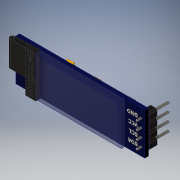
# Autodesk Inventor part: Part1
Saved by Autodesk Inventor 2019 (Build 230136000, 136)
## iProperties
Created: 2025-05-31
Part Number: Part1
Material: Generic
Document SubType Name: Modeling
Designer: Zide
Density: 1 g/cm^3
Appearance: Default
Author: Zide
Autodesk Inventor part; units mm, degrees
(part 1 of 4)
ref_plane "YZ Plane" through (0, 0, 0) normal (1, 0, 0) x (0, 1, 0)
ref_plane "XZ Plane" through (0, 0, 0) normal (0, 1, 0) x (-1, 0, 0)
ref_plane "XY Plane" through (0, 0, 0) normal (0, 0, 1) x (1, 0, 0)
sketch "Sketch1" plane through (0, 0, 0) normal (0, 0, 1) x (1, 0, 0)
  line L0 (-18.8, 6.05) -> (18.8, 6.05)
  line L1 (18.8, -6.05) -> (-18.8, -6.05)
  line L2 (-18.8, -6.05) -> (-18.8, 6.05)
  line L3 (-18.8, 6.05) -> (18.8, -6.05) construction
  line L4 (18.8, 6.05) -> (-18.8, -6.05) construction
  line L5 (-18.8, 0) -> (18.8, 0)
  line L6 (0, 6.05) -> (0, -6.05)
  line L7 (18.8, 3.63) -> (17.8, 3.63)
  line L8 (17.95, 3.38) -> (17.65, 3.38)
  line L9 (17.55, 3.48) -> (17.55, 3.78)
  line L10 (17.65, 3.88) -> (17.95, 3.88)
  line L11 (18.05, 3.78) -> (18.05, 3.48)
  line L12 (18.05, 3.38) -> (17.55, 3.88) construction
  line L13 (17.55, 3.38) -> (18.05, 3.88) construction
  line L14 (17.55, 3.78) -> (17.65, 3.88)
  line L15 (17.95, 3.88) -> (18.05, 3.78)
  line L16 (18.05, 3.48) -> (17.95, 3.38)
  line L17 (17.55, 3.48) -> (17.65, 3.38)
  line L18 (18.8, 1.21) -> (17.8, 1.21)
  line L19 (17.95, 0.96) -> (17.65, 0.96)
  line L20 (17.55, 1.06) -> (17.55, 1.36)
  line L21 (17.65, 1.46) -> (17.95, 1.46)
  line L22 (18.05, 1.36) -> (18.05, 1.06)
  line L23 (18.05, 0.96) -> (17.55, 1.46) construction
  line L24 (17.55, 0.96) -> (18.05, 1.46) construction
  line L25 (17.55, 1.36) -> (17.65, 1.46)
  line L26 (17.95, 1.46) -> (18.05, 1.36)
  line L27 (18.05, 1.06) -> (17.95, 0.96)
  line L28 (17.55, 1.06) -> (17.65, 0.96)
  line L29 (18.8, -1.21) -> (17.8, -1.21)
  line L30 (17.95, -1.46) -> (17.65, -1.46)
  line L31 (17.55, -1.36) -> (17.55, -1.06)
  line L32 (17.65, -0.96) -> (17.95, -0.96)
  line L33 (18.05, -1.06) -> (18.05, -1.36)
  line L34 (18.05, -1.46) -> (17.55, -0.96) construction
  line L35 (17.55, -1.46) -> (18.05, -0.96) construction
  line L36 (17.55, -1.06) -> (17.65, -0.96)
  line L37 (17.95, -0.96) -> (18.05, -1.06)
  line L38 (18.05, -1.36) -> (17.95, -1.46)
  line L39 (17.55, -1.36) -> (17.65, -1.46)
  line L40 (18.8, -3.63) -> (17.8, -3.63)
  line L41 (17.95, -3.88) -> (17.65, -3.88)
  line L42 (17.55, -3.78) -> (17.55, -3.48)
  line L43 (17.65, -3.38) -> (17.95, -3.38)
  line L44 (18.05, -3.48) -> (18.05, -3.78)
  line L45 (18.05, -3.88) -> (17.55, -3.38) construction
  line L46 (17.55, -3.88) -> (18.05, -3.38) construction
  line L47 (17.55, -3.48) -> (17.65, -3.38)
  line L48 (17.95, -3.38) -> (18.05, -3.48)
  line L49 (18.05, -3.78) -> (17.95, -3.88)
  line L50 (17.55, -3.78) -> (17.65, -3.88)
  line L51 (18.8, 3.63) -> (18.8, 1.21)
  line L52 (18.8, 1.21) -> (18.8, -1.21)
  line L53 (18.8, -1.21) -> (18.8, -3.63)
  line L54 (18.8, -6.05) -> (18.8, -3.63)
  line L55 (18.8, 3.63) -> (18.8, 6.05)
  point P0 (0, 0)
  dimension "d0" = 37.6
  dimension "d1" = 12.1
  constraints: 112 end point, 32 point on line, 13 midpoint, 12 equal length, 9 horizontal, 4 perpendicular, 2 vertical
  measures "d0" distance of L0.start L0.end
  measures "d1" distance of L0.end L1.start
extrude "Extrusion1" add sketch "Sketch1" along normal blind 1.1
sketch "Sketch2" plane through (0, 0, 0) normal (0, 0, -1) x (-1, 0, 0)
  line L0 (-17.65, -3.88) -> (-17.95, -3.88)
  line L1 (-17.95, -3.88) -> (-18.05, -3.78)
  line L2 (-18.05, -3.78) -> (-18.05, -3.48)
  line L3 (-18.05, -3.48) -> (-17.95, -3.38)
  line L4 (-17.95, -3.38) -> (-17.65, -3.38)
  line L5 (-17.65, -3.38) -> (-17.55, -3.48)
  line L6 (-17.55, -3.48) -> (-17.55, -3.78)
  line L7 (-17.55, -3.78) -> (-17.65, -3.88)
  line L8 (-17.65, -1.46) -> (-17.95, -1.46)
  line L9 (-17.95, -1.46) -> (-18.05, -1.36)
  line L10 (-18.05, -1.36) -> (-18.05, -1.06)
  line L11 (-18.05, -1.06) -> (-17.95, -0.96)
  line L12 (-17.95, -0.96) -> (-17.65, -0.96)
  line L13 (-17.65, -0.96) -> (-17.55, -1.06)
  line L14 (-17.55, -1.06) -> (-17.55, -1.36)
  line L15 (-17.55, -1.36) -> (-17.65, -1.46)
  line L16 (-17.65, 0.96) -> (-17.95, 0.96)
  line L17 (-17.95, 0.96) -> (-18.05, 1.06)
  line L18 (-18.05, 1.06) -> (-18.05, 1.36)
  line L19 (-18.05, 1.36) -> (-17.95, 1.46)
  line L20 (-17.95, 1.46) -> (-17.65, 1.46)
  line L21 (-17.65, 1.46) -> (-17.55, 1.36)
  line L22 (-17.55, 1.36) -> (-17.55, 1.06)
  line L23 (-17.55, 1.06) -> (-17.65, 0.96)
  line L24 (-17.95, 3.88) -> (-17.65, 3.88)
  line L25 (-17.65, 3.88) -> (-17.55, 3.78)
  line L26 (-17.55, 3.78) -> (-17.55, 3.48)
  line L27 (-17.55, 3.48) -> (-17.65, 3.38)
  line L28 (-17.65, 3.38) -> (-17.95, 3.38)
  line L29 (-17.95, 3.38) -> (-18.05, 3.48)
  line L30 (-18.05, 3.48) -> (-18.05, 3.78)
  line L31 (-18.05, 3.78) -> (-17.95, 3.88)
  line L32 (-18.8, 6.05) -> (18.8, 6.05)
  line L33 (18.8, -6.05) -> (-18.8, -6.05)
  line L34 (18.8, 6.05) -> (18.8, -6.05)
  line L35 (-17.65, 3.38) -> (-17.95, 3.38)
  line L36 (-18.05, 3.78) -> (-18.05, 3.48)
  line L37 (-17.55, 3.48) -> (-17.55, 3.78)
  line L38 (-16.6, -4.33) -> (-16.6, -2.93)
  line L39 (-19, -2.93) -> (-19, -4.33)
  line L40 (-18.5, -4.83) -> (-17.1, -4.83)
  line L41 (-19, -2.93) -> (-18.5, -2.43)
  line L42 (-17.1, -2.43) -> (-16.6, -2.93)
  line L43 (-16.6, -4.33) -> (-17.1, -4.83)
  line L44 (-18.5, -4.83) -> (-19, -4.33)
  line L45 (-16.6, -1.91) -> (-16.6, -0.51)
  line L46 (-19, -0.51) -> (-19, -1.91)
  line L47 (-19, -0.51) -> (-18.5, -0.01)
  line L48 (-17.1, -0.01) -> (-16.6, -0.51)
  line L49 (-16.6, -1.91) -> (-17.1, -2.41)
  line L50 (-18.5, -2.41) -> (-19, -1.91)
  line L51 (-19, 1.91) -> (-18.5, 2.41)
  line L52 (-17.1, 2.41) -> (-16.6, 1.91)
  line L53 (-16.6, 0.51) -> (-16.6, 1.91)
  line L54 (-19, 1.91) -> (-19, 0.51)
  line L55 (-16.6, 0.51) -> (-17.1, 0.01)
  line L56 (-18.5, 0.01) -> (-19, 0.51)
  line L57 (-17.95, 3.88) -> (-17.65, 3.88)
  line L58 (-19, 4.33) -> (-19, 2.93)
  line L59 (-16.6, 2.93) -> (-16.6, 4.33)
  line L60 (-17.1, 4.83) -> (-16.6, 4.33)
  line L61 (-17.1, 4.83) -> (-18.5, 4.83)
  line L62 (-19, 4.33) -> (-18.5, 4.83)
  line L63 (-16.6, 2.93) -> (-17.1, 2.43)
  line L64 (-18.5, 2.43) -> (-19, 2.93)
  line L65 (-18.5, -2.41) -> (-18.5, -2.43)
  line L66 (-17.1, -2.43) -> (-17.1, -2.41)
  line L67 (-18.5, -0.01) -> (-18.5, 0.01)
  line L68 (-17.1, -0.01) -> (-17.1, 0.01)
  line L69 (-18.5, 2.41) -> (-18.5, 2.43)
  line L70 (-17.1, 2.41) -> (-17.1, 2.43)
  point P0 (0, 0)
  constraints: 64 end point, 5 parallel, 5 vertical, 1 perpendicular
extrude "Extrusion2" add sketch "Sketch2" along normal blind 2.3 separate body
sketch "Sketch3" plane through (0, 0, 1.1) normal (0, 0, 1) x (1, 0, 0)
  line L0 (17.95, -3.88) -> (17.65, -3.88)
  line L1 (17.65, -3.88) -> (17.55, -3.78)
  line L2 (17.55, -3.78) -> (17.55, -3.48)
  line L3 (17.55, -3.48) -> (17.65, -3.38)
  line L4 (17.65, -3.38) -> (17.95, -3.38)
  line L5 (17.95, -3.38) -> (18.05, -3.48)
  line L6 (18.05, -3.48) -> (18.05, -3.78)
  line L7 (18.05, -3.78) -> (17.95, -3.88)
  line L8 (17.95, -1.46) -> (17.65, -1.46)
  line L9 (17.65, -1.46) -> (17.55, -1.36)
  line L10 (17.55, -1.36) -> (17.55, -1.06)
  line L11 (17.55, -1.06) -> (17.65, -0.96)
  line L12 (17.65, -0.96) -> (17.95, -0.96)
  line L13 (17.95, -0.96) -> (18.05, -1.06)
  line L14 (18.05, -1.06) -> (18.05, -1.36)
  line L15 (18.05, -1.36) -> (17.95, -1.46)
  line L16 (17.95, 0.96) -> (17.65, 0.96)
  line L17 (17.65, 0.96) -> (17.55, 1.06)
  line L18 (17.55, 1.06) -> (17.55, 1.36)
  line L19 (17.55, 1.36) -> (17.65, 1.46)
  line L20 (17.65, 1.46) -> (17.95, 1.46)
  line L21 (17.95, 1.46) -> (18.05, 1.36)
  line L22 (18.05, 1.36) -> (18.05, 1.06)
  line L23 (18.05, 1.06) -> (17.95, 0.96)
  line L24 (17.65, 3.88) -> (17.95, 3.88)
  line L25 (17.95, 3.88) -> (18.05, 3.78)
  line L26 (18.05, 3.78) -> (18.05, 3.48)
  line L27 (18.05, 3.48) -> (17.95, 3.38)
  line L28 (17.95, 3.38) -> (17.65, 3.38)
  line L29 (17.65, 3.38) -> (17.55, 3.48)
  line L30 (17.55, 3.48) -> (17.55, 3.78)
  line L31 (17.55, 3.78) -> (17.65, 3.88)
  line L32 (18.8, 6.05) -> (-18.8, 6.05)
  line L33 (-18.8, 6.05) -> (-18.8, -6.05)
  line L34 (-18.8, -6.05) -> (18.8, -6.05)
  line L35 (18.8, -6.05) -> (18.8, 6.05)
  point P0 (0, 0)
extrude "Extrusion3" add sketch "Sketch3" along normal blind 1.5 and the other way blind 8 separate body contours L0 L1 L2 L3 L4 L5 L6 L7 | L8 L9 L10 L11 L12 L13 L14 L15 | L16 L17 L18 L19 L20 L21 L22 L23 | L24 L25 L26 L27 L28 L29 L30 L31
chamfer "Chamfer1" distance 0.15 angle 45 32 edges at (18.05, -3.63, 2.6) (17.8, -3.38, 2.6) (17.55, -3.63, 2.6) (17.8, -3.88, 2.6) (18.05, -1.21, 2.6) (17.8, -0.96, 2.6) (17.55, -1.21, 2.6) (17.8, -1.46, 2.6) (18.05, 1.21, 2.6) (17.8, 0.96, 2.6) (17.55, 1.21, 2.6) (17.8, 1.46, 2.6) (17.8, 3.38, 2.6) (18.05, 3.63, 2.6) (17.8, 3.88, 2.6) (17.55, 3.63, 2.6) (17.8, -3.88, -6.9) (18.05, -3.63, -6.9) (17.8, -3.38, -6.9) (17.55, -3.63, -6.9) (17.8, -1.46, -6.9) (17.55, -1.21, -6.9) (17.8, -0.96, -6.9) (18.05, -1.21, -6.9) (17.8, 0.96, -6.9) (17.55, 1.21, -6.9) (17.8, 1.46, -6.9) (18.05, 1.21, -6.9) (17.8, 3.38, -6.9) (17.55, 3.63, -6.9) (17.8, 3.88, -6.9) (18.05, 3.63, -6.9)
sketch "Sketch4" plane through (0, 0, 1.1) normal (0, 0, 1) x (1, 0, 0)
  line L0 (18.8, -6.05) -> (18.8, 6.05)
  line L1 (13, -6.05) -> (13, 6.05)
  line L2 (-14.5, -6.05) -> (-14.5, 6.05)
  line L3 (-11.5, -6.05) -> (-11.5, 6.05)
  line L4 (13, -6.05) -> (-11.5, -6.05)
  line L5 (-11.5, 6.05) -> (13, 6.05)
  line L6 (18.8, 6.05) -> (-18.8, 6.05)
  point P0 (0, 0)
  dimension "d45" = 5.8
  dimension "d46" = 27.5
  dimension "d47" = 3
  constraints: 10 end point, 3 parallel, 1 collinear, 1 perpendicular
  measures "d45" distance between parallel lines of L0 L1
  measures "d46" distance between parallel lines of L1 L2
  measures "d47" distance between parallel lines of L2 L3
extrude "Extrusion4" add sketch "Sketch4" along normal blind 1.5 separate body
sketch "Sketch5" plane through (0, 0, 1.1) normal (0, 0, 1) x (1, 0, 0)
  line L0 (-11.5, 6.05) -> (-11.5, -6.05)
  line L1 (-14.5, 6.05) -> (-14.5, -6.05)
  line L2 (-11.5, -6.05) -> (-14.5, -6.05)
  line L3 (-18.8, -6.05) -> (18.8, -6.05)
  line L4 (-11.5, 6.05) -> (-14.5, 6.05)
  line L5 (18.8, 6.05) -> (-18.8, 6.05)
  point P0 (0, 0)
  dimension "d50" = 3
  constraints: 6 end point, 2 collinear, 1 parallel
  measures "d50" distance between parallel lines of L0 L1
extrude "Extrusion5" add sketch "Sketch5" along normal blind 1.5 separate body
chamfer "Chamfer2" distance 0.5 angle 45 3 edges at (0.75, -6.05, 2.6) (13, 0, 2.6) (0.75, 6.05, 2.6)
sketch "Sketch6" plane through (0, 0, 1.1) normal (0, 0, 1) x (1, 0, 0)
  line L0 (17.55, 3.78) -> (17.55, 3.48)
  line L1 (17.55, 1.36) -> (17.55, 1.06)
  line L2 (17.55, -1.06) -> (17.55, -1.36)
  line L3 (17.55, -3.48) -> (17.55, -3.78)
  line L4 (17.55, -3.48) -> (17.55, -3.78)
  line L5 (17.55, -3.63) -> (16.85, -3.63)
  line L6 (16.819, -4.1169) -> (13.9568, -4.1169) construction
  line L7 (13.9568, -4.1169) -> (13.9568, -3.0812) construction
  line L8 (13.9568, -3.0812) -> (16.819, -3.0812) construction
  line L9 (16.819, -3.0812) -> (16.819, -4.1169) construction
  line L10 (17.55, -1.21) -> (16.85, -1.21)
  line L11 (17.55, 1.21) -> (16.85, 1.21)
  line L12 (17.55, 3.63) -> (16.85, 3.63)
  line L13 (16.8164, -1.7403) -> (14.2403, -1.7403) construction
  line L14 (14.2403, -1.7403) -> (14.2403, -0.7014) construction
  line L15 (14.2403, -0.7014) -> (16.8164, -0.7014) construction
  line L16 (16.8164, -0.7014) -> (16.8164, -1.7403) construction
  line L17 (16.8624, 0.6623) -> (14.0982, 0.6623) construction
  line L18 (14.0982, 0.6623) -> (14.0982, 1.7012) construction
  line L19 (14.0982, 1.7012) -> (16.8624, 1.7012) construction
  line L20 (16.8624, 1.7012) -> (16.8624, 0.6623) construction
  line L21 (16.8549, 3.1406) -> (13.7293, 3.1406) construction
  line L22 (13.7293, 3.1406) -> (13.7293, 4.1811) construction
  line L23 (13.7293, 4.1811) -> (16.8549, 4.1811) construction
  line L24 (16.8549, 4.1811) -> (16.8549, 3.1406) construction
  spline S0 degree 2 poles (16.4065, -3.0812) (16.5216, -3.0812) (16.695, -3.1258) (16.7696, -3.1582) knots 0 0 0 1 2 2 2
  line L25 (16.7696, -3.1582) -> (16.7696, -3.3965)
  line L26 (16.7696, -3.3965) -> (16.7469, -3.3965)
  spline S1 degree 2 poles (16.7469, -3.3965) (16.6715, -3.3325) (16.4908, -3.2636) (16.4057, -3.2636) knots 0 0 0 1 2 2 2
  spline S2 degree 2 poles (16.4057, -3.2636) (16.3838, -3.2636) (16.3133, -3.2733) (16.2923, -3.283) knots 0 0 0 1 2 2 2
  spline S3 degree 2 poles (16.2923, -3.283) (16.2663, -3.2944) (16.2299, -3.3357) (16.2299, -3.3689) knots 0 0 0 1 2 2 2
  spline S4 degree 2 poles (16.2299, -3.3689) (16.2299, -3.407) (16.289, -3.454) (16.3295, -3.4645) knots 0 0 0 1 2 2 2
  spline S5 degree 2 poles (16.3295, -3.4645) (16.3806, -3.4783) (16.4965, -3.5018) (16.5475, -3.5196) knots 0 0 0 1 2 2 2
  spline S6 degree 2 poles (16.5475, -3.5196) (16.6634, -3.5602) (16.7639, -3.6987) (16.7639, -3.8025) knots 0 0 0 1 2 2 2
  spline S7 degree 2 poles (16.7639, -3.8025) (16.7639, -3.9427) (16.5265, -4.1169) (16.3482, -4.1169) knots 0 0 0 1 2 2 2
  spline S8 degree 2 poles (16.3482, -4.1169) (16.259, -4.1169) (16.0824, -4.0804) (16.0127, -4.0496) knots 0 0 0 1 2 2 2
  line L27 (16.0127, -4.0496) -> (16.0127, -3.8211)
  line L28 (16.0127, -3.8211) -> (16.0346, -3.8211)
  spline S9 degree 2 poles (16.0346, -3.8211) (16.0905, -3.8689) (16.2509, -3.9346) (16.3352, -3.9346) knots 0 0 0 1 2 2 2
  spline S10 degree 2 poles (16.3352, -3.9346) (16.3684, -3.9346) (16.4203, -3.9248) (16.4495, -3.9119) knots 0 0 0 1 2 2 2
  spline S11 degree 2 poles (16.4495, -3.9119) (16.473, -3.9013) (16.507, -3.8592) (16.507, -3.8333) knots 0 0 0 1 2 2 2
  spline S12 degree 2 poles (16.507, -3.8333) (16.507, -3.7944) (16.4527, -3.7498) (16.3749, -3.732) knots 0 0 0 1 2 2 2
  spline S13 degree 2 poles (16.3749, -3.732) (16.3247, -3.7206) (16.2315, -3.6987) (16.178, -3.6801) knots 0 0 0 1 2 2 2
  spline S14 degree 2 poles (16.178, -3.6801) (16.0743, -3.642) (15.973, -3.5156) (15.973, -3.4119) knots 0 0 0 1 2 2 2
  spline S15 degree 2 poles (15.973, -3.4119) (15.973, -3.2628) (16.2072, -3.0812) (16.4065, -3.0812) knots 0 0 0 1 2 2 2
  spline S16 degree 2 poles (14.9519, -3.5983) (14.9519, -3.4581) (15.0743, -3.2376) (15.1675, -3.1785) knots 0 0 0 1 2 2 2
  spline S17 degree 2 poles (15.1675, -3.1785) (15.2453, -3.1282) (15.4284, -3.0991) (15.5313, -3.0991) knots 0 0 0 1 2 2 2
  line L29 (15.5313, -3.0991) -> (15.8441, -3.0991)
  line L30 (15.8441, -3.0991) -> (15.8441, -4.0991)
  line L31 (15.8441, -4.0991) -> (15.5346, -4.0991)
  spline S18 degree 2 poles (15.5346, -4.0991) (15.4292, -4.0991) (15.2453, -4.0723) (15.1642, -4.0205) knots 0 0 0 1 2 2 2
  spline S19 degree 2 poles (15.1642, -4.0205) (15.0662, -3.9572) (14.9519, -3.7433) (14.9519, -3.5983) knots 0 0 0 1 2 2 2
  spline S20 degree 2 poles (15.2096, -3.5999) (15.2096, -3.6987) (15.2777, -3.8397) (15.3474, -3.8795) knots 0 0 0 1 2 2 2
  spline S21 degree 2 poles (15.3474, -3.8795) (15.3984, -3.907) (15.5103, -3.9127) (15.588, -3.9127) knots 0 0 0 1 2 2 2
  line L32 (15.588, -3.9127) -> (15.5929, -3.9127)
  line L33 (15.5929, -3.9127) -> (15.5929, -3.2863)
  line L34 (15.5929, -3.2863) -> (15.588, -3.2863)
  spline S22 degree 2 poles (15.588, -3.2863) (15.5038, -3.2863) (15.3879, -3.2919) (15.3352, -3.3252) knots 0 0 0 1 2 2 2
  spline S23 degree 2 poles (15.3352, -3.3252) (15.2736, -3.3641) (15.2096, -3.501) (15.2096, -3.5999) knots 0 0 0 1 2 2 2
  line L35 (14.9106, -3.0991) -> (14.5727, -4.0991)
  line L36 (14.5727, -4.0991) -> (14.2987, -4.0991)
  line L37 (14.2987, -4.0991) -> (13.9608, -3.0991)
  line L38 (13.9608, -3.0991) -> (14.2193, -3.0991)
  line L39 (14.2193, -3.0991) -> (14.2817, -3.3033)
  line L40 (14.2817, -3.3033) -> (14.5962, -3.3033)
  line L41 (14.5962, -3.3033) -> (14.6594, -3.0991)
  line L42 (14.6594, -3.0991) -> (14.9106, -3.0991)
  line L43 (14.3368, -3.4848) -> (14.4389, -3.8154)
  line L44 (14.4389, -3.8154) -> (14.5419, -3.4848)
  line L45 (14.5419, -3.4848) -> (14.3368, -3.4848)
  spline S24 degree 2 poles (16.404, -0.703) (16.519, -0.703) (16.6925, -0.7476) (16.767, -0.78) knots 0 0 0 1 2 2 2
  line L46 (16.767, -0.78) -> (16.767, -1.0183)
  line L47 (16.767, -1.0183) -> (16.7443, -1.0183)
  spline S25 degree 2 poles (16.7443, -1.0183) (16.669, -0.9543) (16.4882, -0.8854) (16.4032, -0.8854) knots 0 0 0 1 2 2 2
  spline S26 degree 2 poles (16.4032, -0.8854) (16.3813, -0.8854) (16.3108, -0.8951) (16.2897, -0.9048) knots 0 0 0 1 2 2 2
  spline S27 degree 2 poles (16.2897, -0.9048) (16.2638, -0.9162) (16.2273, -0.9575) (16.2273, -0.9907) knots 0 0 0 1 2 2 2
  spline S28 degree 2 poles (16.2273, -0.9907) (16.2273, -1.0288) (16.2865, -1.0758) (16.327, -1.0863) knots 0 0 0 1 2 2 2
  spline S29 degree 2 poles (16.327, -1.0863) (16.378, -1.1001) (16.4939, -1.1236) (16.545, -1.1415) knots 0 0 0 1 2 2 2
  spline S30 degree 2 poles (16.545, -1.1415) (16.6609, -1.182) (16.7613, -1.3205) (16.7613, -1.4243) knots 0 0 0 1 2 2 2
  spline S31 degree 2 poles (16.7613, -1.4243) (16.7613, -1.5645) (16.5239, -1.7387) (16.3456, -1.7387) knots 0 0 0 1 2 2 2
  spline S32 degree 2 poles (16.3456, -1.7387) (16.2565, -1.7387) (16.0798, -1.7022) (16.0101, -1.6714) knots 0 0 0 1 2 2 2
  line L48 (16.0101, -1.6714) -> (16.0101, -1.4429)
  line L49 (16.0101, -1.4429) -> (16.032, -1.4429)
  spline S33 degree 2 poles (16.032, -1.4429) (16.0879, -1.4907) (16.2484, -1.5564) (16.3327, -1.5564) knots 0 0 0 1 2 2 2
  spline S34 degree 2 poles (16.3327, -1.5564) (16.3659, -1.5564) (16.4177, -1.5466) (16.4469, -1.5337) knots 0 0 0 1 2 2 2
  spline S35 degree 2 poles (16.4469, -1.5337) (16.4704, -1.5231) (16.5045, -1.481) (16.5045, -1.4551) knots 0 0 0 1 2 2 2
  spline S36 degree 2 poles (16.5045, -1.4551) (16.5045, -1.4162) (16.4502, -1.3716) (16.3724, -1.3538) knots 0 0 0 1 2 2 2
  spline S37 degree 2 poles (16.3724, -1.3538) (16.3221, -1.3424) (16.2289, -1.3205) (16.1754, -1.3019) knots 0 0 0 1 2 2 2
  spline S38 degree 2 poles (16.1754, -1.3019) (16.0717, -1.2638) (15.9704, -1.1374) (15.9704, -1.0337) knots 0 0 0 1 2 2 2
  spline S39 degree 2 poles (15.9704, -1.0337) (15.9704, -0.8846) (16.2046, -0.703) (16.404, -0.703) knots 0 0 0 1 2 2 2
  spline S40 degree 2 poles (15.4104, -0.7014) (15.6357, -0.7014) (15.8999, -0.9737) (15.8999, -1.2201) knots 0 0 0 1 2 2 2
  spline S41 degree 2 poles (15.8999, -1.2201) (15.8999, -1.4575) (15.6349, -1.7403) (15.4096, -1.7403) knots 0 0 0 1 2 2 2
  spline S42 degree 2 poles (15.4096, -1.7403) (15.3505, -1.7403) (15.2549, -1.7265) (15.2111, -1.7152) knots 0 0 0 1 2 2 2
  spline S43 degree 2 poles (15.2111, -1.7152) (15.1771, -1.7047) (15.0968, -1.6698) (15.0717, -1.6568) knots 0 0 0 1 2 2 2
  line L50 (15.0717, -1.6568) -> (15.0717, -1.4186)
  line L51 (15.0717, -1.4186) -> (15.0968, -1.4186)
  spline S44 degree 2 poles (15.0968, -1.4186) (15.1155, -1.4348) (15.1706, -1.4802) (15.2054, -1.5013) knots 0 0 0 1 2 2 2
  spline S45 degree 2 poles (15.2054, -1.5013) (15.2403, -1.5231) (15.3237, -1.5531) (15.3699, -1.5531) knots 0 0 0 1 2 2 2
  spline S46 degree 2 poles (15.3699, -1.5531) (15.4242, -1.5531) (15.5142, -1.5191) (15.5555, -1.4761) knots 0 0 0 1 2 2 2
  spline S47 degree 2 poles (15.5555, -1.4761) (15.5928, -1.438) (15.6406, -1.3076) (15.6406, -1.2192) knots 0 0 0 1 2 2 2
  spline S48 degree 2 poles (15.6406, -1.2192) (15.6406, -1.1261) (15.5912, -0.9988) (15.5506, -0.9599) knots 0 0 0 1 2 2 2
  spline S49 degree 2 poles (15.5506, -0.9599) (15.5117, -0.9218) (15.4161, -0.8886) (15.3683, -0.8886) knots 0 0 0 1 2 2 2
  spline S50 degree 2 poles (15.3683, -0.8886) (15.3189, -0.8886) (15.2289, -0.9218) (15.1981, -0.9421) knots 0 0 0 1 2 2 2
  spline S51 degree 2 poles (15.1981, -0.9421) (15.1641, -0.9624) (15.113, -1.0053) (15.0944, -1.0223) knots 0 0 0 1 2 2 2
  line L52 (15.0944, -1.0223) -> (15.0717, -1.0223)
  line L53 (15.0717, -1.0223) -> (15.0717, -0.7873)
  spline S52 degree 2 poles (15.0717, -0.7873) (15.0993, -0.7744) (15.1714, -0.7419) (15.2103, -0.7306) knots 0 0 0 1 2 2 2
  spline S53 degree 2 poles (15.2103, -0.7306) (15.2573, -0.716) (15.3391, -0.7014) (15.4104, -0.7014) knots 0 0 0 1 2 2 2
  line L54 (14.2565, -0.7209) -> (14.9234, -0.7209)
  line L55 (14.9234, -0.7209) -> (14.9234, -1.7209)
  line L56 (14.9234, -1.7209) -> (14.6722, -1.7209)
  line L57 (14.6722, -1.7209) -> (14.6722, -0.9113)
  line L58 (14.6722, -0.9113) -> (14.2565, -0.9113)
  line L59 (14.2565, -0.9113) -> (14.2565, -0.7209)
  line L60 (15.924, 0.6818) -> (16.2676, 1.6818)
  line L61 (16.2676, 1.6818) -> (16.5293, 1.6818)
  line L62 (16.5293, 1.6818) -> (16.8729, 0.6818)
  line L63 (16.8729, 0.6818) -> (16.6128, 0.6818)
  line L64 (16.6128, 0.6818) -> (16.3948, 1.3601)
  line L65 (16.3948, 1.3601) -> (16.1776, 0.6818)
  line L66 (16.1776, 0.6818) -> (15.924, 0.6818)
  spline S54 degree 2 poles (15.3997, 1.7012) (15.6249, 1.7012) (15.8891, 1.4289) (15.8891, 1.1826) knots 0 0 0 1 2 2 2
  spline S55 degree 2 poles (15.8891, 1.1826) (15.8891, 0.9451) (15.6241, 0.6623) (15.3988, 0.6623) knots 0 0 0 1 2 2 2
  spline S56 degree 2 poles (15.3988, 0.6623) (15.3397, 0.6623) (15.2441, 0.6761) (15.2003, 0.6875) knots 0 0 0 1 2 2 2
  spline S57 degree 2 poles (15.2003, 0.6875) (15.1663, 0.698) (15.086, 0.7328) (15.0609, 0.7458) knots 0 0 0 1 2 2 2
  line L67 (15.0609, 0.7458) -> (15.0609, 0.984)
  line L68 (15.0609, 0.984) -> (15.086, 0.984)
  spline S58 degree 2 poles (15.086, 0.984) (15.1047, 0.9678) (15.1598, 0.9225) (15.1946, 0.9014) knots 0 0 0 1 2 2 2
  spline S59 degree 2 poles (15.1946, 0.9014) (15.2295, 0.8795) (15.3129, 0.8495) (15.3591, 0.8495) knots 0 0 0 1 2 2 2
  spline S60 degree 2 poles (15.3591, 0.8495) (15.4134, 0.8495) (15.5034, 0.8836) (15.5447, 0.9265) knots 0 0 0 1 2 2 2
  spline S61 degree 2 poles (15.5447, 0.9265) (15.582, 0.9646) (15.6298, 1.0951) (15.6298, 1.1834) knots 0 0 0 1 2 2 2
  spline S62 degree 2 poles (15.6298, 1.1834) (15.6298, 1.2766) (15.5804, 1.4038) (15.5399, 1.4427) knots 0 0 0 1 2 2 2
  spline S63 degree 2 poles (15.5399, 1.4427) (15.501, 1.4808) (15.4053, 1.514) (15.3575, 1.514) knots 0 0 0 1 2 2 2
  spline S64 degree 2 poles (15.3575, 1.514) (15.3081, 1.514) (15.2181, 1.4808) (15.1873, 1.4605) knots 0 0 0 1 2 2 2
  spline S65 degree 2 poles (15.1873, 1.4605) (15.1533, 1.4403) (15.1023, 1.3973) (15.0836, 1.3803) knots 0 0 0 1 2 2 2
  line L69 (15.0836, 1.3803) -> (15.0609, 1.3803)
  line L70 (15.0609, 1.3803) -> (15.0609, 1.6153)
  spline S66 degree 2 poles (15.0609, 1.6153) (15.0885, 1.6283) (15.1606, 1.6607) (15.1995, 1.6721) knots 0 0 0 1 2 2 2
  spline S67 degree 2 poles (15.1995, 1.6721) (15.2465, 1.6866) (15.3283, 1.7012) (15.3997, 1.7012) knots 0 0 0 1 2 2 2
  spline S68 degree 2 poles (14.4815, 1.7012) (14.7068, 1.7012) (14.971, 1.4289) (14.971, 1.1826) knots 0 0 0 1 2 2 2
  spline S69 degree 2 poles (14.971, 1.1826) (14.971, 0.9451) (14.706, 0.6623) (14.4807, 0.6623) knots 0 0 0 1 2 2 2
  spline S70 degree 2 poles (14.4807, 0.6623) (14.4215, 0.6623) (14.3259, 0.6761) (14.2822, 0.6875) knots 0 0 0 1 2 2 2
  spline S71 degree 2 poles (14.2822, 0.6875) (14.2481, 0.698) (14.1679, 0.7328) (14.1428, 0.7458) knots 0 0 0 1 2 2 2
  line L71 (14.1428, 0.7458) -> (14.1428, 0.984)
  line L72 (14.1428, 0.984) -> (14.1679, 0.984)
  spline S72 degree 2 poles (14.1679, 0.984) (14.1865, 0.9678) (14.2416, 0.9225) (14.2765, 0.9014) knots 0 0 0 1 2 2 2
  spline S73 degree 2 poles (14.2765, 0.9014) (14.3113, 0.8795) (14.3948, 0.8495) (14.441, 0.8495) knots 0 0 0 1 2 2 2
  spline S74 degree 2 poles (14.441, 0.8495) (14.4953, 0.8495) (14.5852, 0.8836) (14.6266, 0.9265) knots 0 0 0 1 2 2 2
  spline S75 degree 2 poles (14.6266, 0.9265) (14.6638, 0.9646) (14.7117, 1.0951) (14.7117, 1.1834) knots 0 0 0 1 2 2 2
  spline S76 degree 2 poles (14.7117, 1.1834) (14.7117, 1.2766) (14.6622, 1.4038) (14.6217, 1.4427) knots 0 0 0 1 2 2 2
  spline S77 degree 2 poles (14.6217, 1.4427) (14.5828, 1.4808) (14.4872, 1.514) (14.4394, 1.514) knots 0 0 0 1 2 2 2
  spline S78 degree 2 poles (14.4394, 1.514) (14.3899, 1.514) (14.3, 1.4808) (14.2692, 1.4605) knots 0 0 0 1 2 2 2
  spline S79 degree 2 poles (14.2692, 1.4605) (14.2352, 1.4403) (14.1841, 1.3973) (14.1655, 1.3803) knots 0 0 0 1 2 2 2
  line L73 (14.1655, 1.3803) -> (14.1428, 1.3803)
  line L74 (14.1428, 1.3803) -> (14.1428, 1.6153)
  spline S80 degree 2 poles (14.1428, 1.6153) (14.1703, 1.6283) (14.2424, 1.6607) (14.2813, 1.6721) knots 0 0 0 1 2 2 2
  spline S81 degree 2 poles (14.2813, 1.6721) (14.3283, 1.6866) (14.4102, 1.7012) (14.4815, 1.7012) knots 0 0 0 1 2 2 2
  spline S82 degree 2 poles (15.9165, 4.1033) (15.9821, 4.13) (16.192, 4.1811) (16.2941, 4.1811) knots 0 0 0 1 2 2 2
  spline S83 degree 2 poles (16.2941, 4.1811) (16.53, 4.1811) (16.8095, 3.9088) (16.8095, 3.6592) knots 0 0 0 1 2 2 2
  spline S84 degree 2 poles (16.8095, 3.6592) (16.8095, 3.4242) (16.53, 3.1406) (16.2868, 3.1406) knots 0 0 0 1 2 2 2
  spline S85 degree 2 poles (16.2868, 3.1406) (16.1612, 3.1406) (16.004, 3.1884) (15.9206, 3.2289) knots 0 0 0 1 2 2 2
  line L75 (15.9206, 3.2289) -> (15.9206, 3.4639)
  line L76 (15.9206, 3.4639) -> (15.9432, 3.4639)
  spline S86 degree 2 poles (15.9432, 3.4639) (15.9611, 3.4501) (16.0291, 3.3975) (16.0616, 3.3796) knots 0 0 0 1 2 2 2
  spline S87 degree 2 poles (16.0616, 3.3796) (16.0988, 3.3578) (16.1977, 3.327) (16.2528, 3.327) knots 0 0 0 1 2 2 2
  spline S88 degree 2 poles (16.2528, 3.327) (16.3168, 3.327) (16.423, 3.3675) (16.4643, 3.4088) knots 0 0 0 1 2 2 2
  spline S89 degree 2 poles (16.4643, 3.4088) (16.504, 3.4493) (16.5502, 3.5733) (16.5502, 3.6552) knots 0 0 0 1 2 2 2
  spline S90 degree 2 poles (16.5502, 3.6552) (16.5502, 3.8302) (16.3744, 3.9971) (16.2228, 3.9971) knots 0 0 0 1 2 2 2
  spline S91 degree 2 poles (16.2228, 3.9971) (16.209, 3.9971) (16.1734, 3.9955) (16.1596, 3.9947) knots 0 0 0 1 2 2 2
  line L77 (16.1596, 3.9947) -> (16.1596, 3.7978)
  line L78 (16.1596, 3.7978) -> (16.3533, 3.7978)
  line L79 (16.3533, 3.7978) -> (16.3533, 3.6106)
  line L80 (16.3533, 3.6106) -> (15.9165, 3.6106)
  line L81 (15.9165, 3.6106) -> (15.9165, 4.1033)
  line L82 (14.8703, 4.16) -> (15.1118, 4.16)
  line L83 (15.1118, 4.16) -> (15.4975, 3.4631)
  line L84 (15.4975, 3.4631) -> (15.4975, 4.16)
  line L85 (15.4975, 4.16) -> (15.7269, 4.16)
  line L86 (15.7269, 4.16) -> (15.7269, 3.16)
  line L87 (15.7269, 3.16) -> (15.4189, 3.16)
  line L88 (15.4189, 3.16) -> (15.0996, 3.733)
  line L89 (15.0996, 3.733) -> (15.0996, 3.16)
  line L90 (15.0996, 3.16) -> (14.8703, 3.16)
  line L91 (14.8703, 3.16) -> (14.8703, 4.16)
  spline S92 degree 2 poles (13.7747, 3.6608) (13.7747, 3.801) (13.8971, 4.0214) (13.9902, 4.0806) knots 0 0 0 1 2 2 2
  spline S93 degree 2 poles (13.9902, 4.0806) (14.068, 4.1308) (14.2512, 4.16) (14.3541, 4.16) knots 0 0 0 1 2 2 2
  line L92 (14.3541, 4.16) -> (14.6669, 4.16)
  line L93 (14.6669, 4.16) -> (14.6669, 3.16)
  line L94 (14.6669, 3.16) -> (14.3573, 3.16)
  spline S94 degree 2 poles (14.3573, 3.16) (14.252, 3.16) (14.068, 3.1868) (13.987, 3.2386) knots 0 0 0 1 2 2 2
  spline S95 degree 2 poles (13.987, 3.2386) (13.8889, 3.3018) (13.7747, 3.5158) (13.7747, 3.6608) knots 0 0 0 1 2 2 2
  spline S96 degree 2 poles (14.0324, 3.6592) (14.0324, 3.5603) (14.1005, 3.4193) (14.1701, 3.3796) knots 0 0 0 1 2 2 2
  spline S97 degree 2 poles (14.1701, 3.3796) (14.2212, 3.3521) (14.333, 3.3464) (14.4108, 3.3464) knots 0 0 0 1 2 2 2
  line L95 (14.4108, 3.3464) -> (14.4157, 3.3464)
  line L96 (14.4157, 3.3464) -> (14.4157, 3.9728)
  line L97 (14.4157, 3.9728) -> (14.4108, 3.9728)
  spline S98 degree 2 poles (14.4108, 3.9728) (14.3265, 3.9728) (14.2107, 3.9672) (14.158, 3.9339) knots 0 0 0 1 2 2 2
  spline S99 degree 2 poles (14.158, 3.9339) (14.0964, 3.895) (14.0324, 3.7581) (14.0324, 3.6592) knots 0 0 0 1 2 2 2
  point P0 (0, 0)
  dimension "d56" = 0.7
  dimension "d57" = 0.7
  dimension "d58" = 0.7
  dimension "d59" = 0.7
  constraints: 8 end point, 4 horizontal, 1 midpoint, 8 other
  measures "d56" distance of L5.start L5.end
  measures "d57" distance of L10.start L10.end
  measures "d58" distance of L11.start L11.end
  measures "d59" distance of L12.start L12.end
extrude "Extrusion6" add sketch "Sketch6" along normal blind 0.1 separate body
sketch "Sketch7" plane through (0, 0, 2.6) normal (0, 0, 1) x (1, 0, 0)
  line L0 (-13.8224, -5.7117) -> (-13.8224, 3.2469) construction
  line L1 (-13.8224, 3.2469) -> (-12.7802, 3.2469) construction
  line L2 (-12.7802, 3.2469) -> (-12.7802, -5.7117) construction
  line L3 (-12.7802, -5.7117) -> (-13.8224, -5.7117) construction
  line L4 (-13.7908, -3.8787) -> (-12.2908, -4.2555)
  line L5 (-12.2908, -4.2555) -> (-12.2908, -4.4792)
  line L6 (-12.2908, -4.4792) -> (-13.5355, -4.7843)
  line L7 (-13.5355, -4.7843) -> (-12.2908, -5.0809)
  line L8 (-12.2908, -5.0809) -> (-12.2908, -5.3021)
  line L9 (-12.2908, -5.3021) -> (-13.7908, -5.685)
  line L10 (-13.7908, -5.685) -> (-13.7908, -5.4796)
  line L11 (-13.7908, -5.4796) -> (-12.5473, -5.1781)
  line L12 (-12.5473, -5.1781) -> (-13.7908, -4.8791)
  line L13 (-13.7908, -4.8791) -> (-13.7908, -4.6761)
  line L14 (-13.7908, -4.6761) -> (-12.5327, -4.3746)
  line L15 (-12.5327, -4.3746) -> (-13.7908, -4.0744)
  line L16 (-13.7908, -4.0744) -> (-13.7908, -3.8787)
  line L17 (-13.7908, -2.0189) -> (-12.2908, -2.3957)
  line L18 (-12.2908, -2.3957) -> (-12.2908, -2.6193)
  line L19 (-12.2908, -2.6193) -> (-13.5355, -2.9245)
  line L20 (-13.5355, -2.9245) -> (-12.2908, -3.221)
  line L21 (-12.2908, -3.221) -> (-12.2908, -3.4423)
  line L22 (-12.2908, -3.4423) -> (-13.7908, -3.8252)
  line L23 (-13.7908, -3.8252) -> (-13.7908, -3.6198)
  line L24 (-13.7908, -3.6198) -> (-12.5473, -3.3183)
  line L25 (-12.5473, -3.3183) -> (-13.7908, -3.0193)
  line L26 (-13.7908, -3.0193) -> (-13.7908, -2.8163)
  line L27 (-13.7908, -2.8163) -> (-12.5327, -2.5148)
  line L28 (-12.5327, -2.5148) -> (-13.7908, -2.2146)
  line L29 (-13.7908, -2.2146) -> (-13.7908, -2.0189)
  line L30 (-12.2908, -0.9577) -> (-12.2908, -1.8827)
  line L31 (-12.2908, -1.8827) -> (-12.5035, -1.8827)
  spline S0 degree 2 poles (-12.5035, -1.8827) (-12.5971, -1.783) (-12.7709, -1.6056) (-12.8645, -1.5205) knots 0 0 0 1 2 2 2
  spline S1 degree 2 poles (-12.8645, -1.5205) (-13.0529, -1.3491) (-13.279, -1.2239) (-13.3994, -1.2239) knots 0 0 0 1 2 2 2
  spline S2 degree 2 poles (-13.3994, -1.2239) (-13.4626, -1.2239) (-13.5574, -1.2628) (-13.5878, -1.298) knots 0 0 0 1 2 2 2
  spline S3 degree 2 poles (-13.5878, -1.298) (-13.6182, -1.3333) (-13.6486, -1.4257) (-13.6486, -1.4816) knots 0 0 0 1 2 2 2
  spline S4 degree 2 poles (-13.6486, -1.4816) (-13.6486, -1.5351) (-13.6218, -1.6445) (-13.6012, -1.6943) knots 0 0 0 1 2 2 2
  spline S5 degree 2 poles (-13.6012, -1.6943) (-13.5841, -1.7369) (-13.5355, -1.8159) (-13.5185, -1.8402) knots 0 0 0 1 2 2 2
  line L32 (-13.5185, -1.8402) -> (-13.5185, -1.8511)
  line L33 (-13.5185, -1.8511) -> (-13.7324, -1.8511)
  spline S6 degree 2 poles (-13.7324, -1.8511) (-13.7628, -1.7891) (-13.8224, -1.5667) (-13.8224, -1.467) knots 0 0 0 1 2 2 2
  spline S7 degree 2 poles (-13.8224, -1.467) (-13.8224, -1.2567) (-13.5999, -1.0197) (-13.4103, -1.0197) knots 0 0 0 1 2 2 2
  spline S8 degree 2 poles (-13.4103, -1.0197) (-13.3216, -1.0197) (-13.1733, -1.061) (-13.1101, -1.0975) knots 0 0 0 1 2 2 2
  spline S9 degree 2 poles (-13.1101, -1.0975) (-13.0444, -1.1339) (-12.9156, -1.2397) (-12.8536, -1.298) knots 0 0 0 1 2 2 2
  spline S10 degree 2 poles (-12.8536, -1.298) (-12.7503, -1.3928) (-12.529, -1.625) (-12.4646, -1.6943) knots 0 0 0 1 2 2 2
  line L34 (-12.4646, -1.6943) -> (-12.4646, -0.9577)
  line L35 (-12.4646, -0.9577) -> (-12.2908, -0.9577)
  spline S11 degree 2 poles (-13.6486, -0.3523) (-13.6486, -0.407) (-13.6218, -0.5152) (-13.6012, -0.5675) knots 0 0 0 1 2 2 2
  spline S12 degree 2 poles (-13.6012, -0.5675) (-13.5805, -0.6161) (-13.5367, -0.6878) (-13.5173, -0.7158) knots 0 0 0 1 2 2 2
  line L36 (-13.5173, -0.7158) -> (-13.5173, -0.7279)
  line L37 (-13.5173, -0.7279) -> (-13.73, -0.7279)
  spline S13 degree 2 poles (-13.73, -0.7279) (-13.7653, -0.6623) (-13.8224, -0.4374) (-13.8224, -0.3365) knots 0 0 0 1 2 2 2
  spline S14 degree 2 poles (-13.8224, -0.3365) (-13.8224, -0.2344) (-13.7811, -0.0825) (-13.7373, -0.0205) knots 0 0 0 1 2 2 2
  spline S15 degree 2 poles (-13.7373, -0.0205) (-13.6899, 0.0452) (-13.5525, 0.1132) (-13.4602, 0.1132) knots 0 0 0 1 2 2 2
  spline S16 degree 2 poles (-13.4602, 0.1132) (-13.3362, 0.1132) (-13.149, -0.0497) (-13.1247, -0.1639) knots 0 0 0 1 2 2 2
  line L38 (-13.1247, -0.1639) -> (-13.1101, -0.1639)
  spline S17 degree 2 poles (-13.1101, -0.1639) (-13.1003, -0.1165) (-13.0566, -0.0083) (-13.0128, 0.0379) knots 0 0 0 1 2 2 2
  spline S18 degree 2 poles (-13.0128, 0.0379) (-12.9703, 0.0841) (-12.8341, 0.1424) (-12.7357, 0.1424) knots 0 0 0 1 2 2 2
  spline S19 degree 2 poles (-12.7357, 0.1424) (-12.6348, 0.1424) (-12.4634, 0.0731) (-12.3978, 0.0099) knots 0 0 0 1 2 2 2
  spline S20 degree 2 poles (-12.3978, 0.0099) (-12.3297, -0.0557) (-12.2592, -0.2417) (-12.2592, -0.3596) knots 0 0 0 1 2 2 2
  spline S21 degree 2 poles (-12.2592, -0.3596) (-12.2592, -0.4727) (-12.3139, -0.6939) (-12.3516, -0.7693) knots 0 0 0 1 2 2 2
  line L39 (-12.3516, -0.7693) -> (-12.5643, -0.7693)
  line L40 (-12.5643, -0.7693) -> (-12.5643, -0.7547)
  spline S22 degree 2 poles (-12.5643, -0.7547) (-12.5181, -0.6915) (-12.433, -0.4775) (-12.433, -0.3718) knots 0 0 0 1 2 2 2
  spline S23 degree 2 poles (-12.433, -0.3718) (-12.433, -0.3098) (-12.4719, -0.1858) (-12.5169, -0.1445) knots 0 0 0 1 2 2 2
  spline S24 degree 2 poles (-12.5169, -0.1445) (-12.5619, -0.1044) (-12.6688, -0.0618) (-12.7503, -0.0618) knots 0 0 0 1 2 2 2
  spline S25 degree 2 poles (-12.7503, -0.0618) (-12.8317, -0.0618) (-12.9375, -0.1092) (-12.9679, -0.1518) knots 0 0 0 1 2 2 2
  spline S26 degree 2 poles (-12.9679, -0.1518) (-12.9982, -0.1943) (-13.0213, -0.3098) (-13.0213, -0.3779) knots 0 0 0 1 2 2 2
  line L41 (-13.0213, -0.3779) -> (-13.0213, -0.4629)
  line L42 (-13.0213, -0.4629) -> (-13.1879, -0.4629)
  line L43 (-13.1879, -0.4629) -> (-13.1879, -0.3961)
  spline S27 degree 2 poles (-13.1879, -0.3961) (-13.1879, -0.2612) (-13.3167, -0.091) (-13.4395, -0.091) knots 0 0 0 1 2 2 2
  spline S28 degree 2 poles (-13.4395, -0.091) (-13.4966, -0.091) (-13.5781, -0.1347) (-13.6024, -0.17) knots 0 0 0 1 2 2 2
  spline S29 degree 2 poles (-13.6024, -0.17) (-13.6279, -0.2077) (-13.6486, -0.3001) (-13.6486, -0.3523) knots 0 0 0 1 2 2 2
  spline S30 degree 2 poles (-13.0408, 1.302) (-12.6372, 1.302) (-12.2592, 1.0674) (-12.2592, 0.8231) knots 0 0 0 1 2 2 2
  spline S31 degree 2 poles (-12.2592, 0.8231) (-12.2592, 0.5751) (-12.6445, 0.343) (-13.0396, 0.343) knots 0 0 0 1 2 2 2
  spline S32 degree 2 poles (-13.0396, 0.343) (-13.4456, 0.343) (-13.8212, 0.5776) (-13.8212, 0.8231) knots 0 0 0 1 2 2 2
  spline S33 degree 2 poles (-13.8212, 0.8231) (-13.8212, 1.0699) (-13.4322, 1.302) (-13.0408, 1.302) knots 0 0 0 1 2 2 2
  spline S34 degree 2 poles (-12.5837, 1.0443) (-12.6579, 1.0735) (-12.8864, 1.0978) (-13.0408, 1.0978) knots 0 0 0 1 2 2 2
  spline S35 degree 2 poles (-13.0408, 1.0978) (-13.1952, 1.0978) (-13.4225, 1.0735) (-13.4991, 1.0431) knots 0 0 0 1 2 2 2
  spline S36 degree 2 poles (-13.4991, 1.0431) (-13.5756, 1.0127) (-13.6546, 0.907) (-13.6546, 0.8231) knots 0 0 0 1 2 2 2
  spline S37 degree 2 poles (-13.6546, 0.8231) (-13.6546, 0.7392) (-13.5756, 0.6311) (-13.4966, 0.5995) knots 0 0 0 1 2 2 2
  spline S38 degree 2 poles (-13.4966, 0.5995) (-13.42, 0.5691) (-13.1867, 0.5472) (-13.0396, 0.5472) knots 0 0 0 1 2 2 2
  spline S39 degree 2 poles (-13.0396, 0.5472) (-12.8815, 0.5472) (-12.67, 0.5666) (-12.5874, 0.5982) knots 0 0 0 1 2 2 2
  spline S40 degree 2 poles (-12.5874, 0.5982) (-12.5096, 0.6274) (-12.4257, 0.7356) (-12.4257, 0.8231) knots 0 0 0 1 2 2 2
  spline S41 degree 2 poles (-12.4257, 0.8231) (-12.4257, 0.9058) (-12.5047, 1.014) (-12.5837, 1.0443) knots 0 0 0 1 2 2 2
  line L44 (-12.2908, 2.4191) -> (-12.2908, 1.4941)
  line L45 (-12.2908, 1.4941) -> (-12.5035, 1.4941)
  spline S42 degree 2 poles (-12.5035, 1.4941) (-12.5971, 1.5938) (-12.7709, 1.7713) (-12.8645, 1.8563) knots 0 0 0 1 2 2 2
  spline S43 degree 2 poles (-12.8645, 1.8563) (-13.0529, 2.0277) (-13.279, 2.1529) (-13.3994, 2.1529) knots 0 0 0 1 2 2 2
  spline S44 degree 2 poles (-13.3994, 2.1529) (-13.4626, 2.1529) (-13.5574, 2.114) (-13.5878, 2.0788) knots 0 0 0 1 2 2 2
  spline S45 degree 2 poles (-13.5878, 2.0788) (-13.6182, 2.0435) (-13.6486, 1.9512) (-13.6486, 1.8952) knots 0 0 0 1 2 2 2
  spline S46 degree 2 poles (-13.6486, 1.8952) (-13.6486, 1.8418) (-13.6218, 1.7324) (-13.6012, 1.6825) knots 0 0 0 1 2 2 2
  spline S47 degree 2 poles (-13.6012, 1.6825) (-13.5841, 1.64) (-13.5355, 1.561) (-13.5185, 1.5366) knots 0 0 0 1 2 2 2
  line L46 (-13.5185, 1.5366) -> (-13.5185, 1.5257)
  line L47 (-13.5185, 1.5257) -> (-13.7324, 1.5257)
  spline S48 degree 2 poles (-13.7324, 1.5257) (-13.7628, 1.5877) (-13.8224, 1.8101) (-13.8224, 1.9098) knots 0 0 0 1 2 2 2
  spline S49 degree 2 poles (-13.8224, 1.9098) (-13.8224, 2.1201) (-13.5999, 2.3572) (-13.4103, 2.3572) knots 0 0 0 1 2 2 2
  spline S50 degree 2 poles (-13.4103, 2.3572) (-13.3216, 2.3572) (-13.1733, 2.3158) (-13.1101, 2.2794) knots 0 0 0 1 2 2 2
  spline S51 degree 2 poles (-13.1101, 2.2794) (-13.0444, 2.2429) (-12.9156, 2.1371) (-12.8536, 2.0788) knots 0 0 0 1 2 2 2
  spline S52 degree 2 poles (-12.8536, 2.0788) (-12.7503, 1.984) (-12.529, 1.7518) (-12.4646, 1.6825) knots 0 0 0 1 2 2 2
  line L48 (-12.4646, 1.6825) -> (-12.4646, 2.4191)
  line L49 (-12.4646, 2.4191) -> (-12.2908, 2.4191)
  spline S53 degree 2 poles (-13.3033, 2.5784) (-13.4188, 2.5784) (-13.6109, 2.6537) (-13.6802, 2.7194) knots 0 0 0 1 2 2 2
  spline S54 degree 2 poles (-13.6802, 2.7194) (-13.747, 2.7814) (-13.8212, 2.9625) (-13.8212, 3.0549) knots 0 0 0 1 2 2 2
  spline S55 degree 2 poles (-13.8212, 3.0549) (-13.8212, 3.1582) (-13.7519, 3.326) (-13.6862, 3.3879) knots 0 0 0 1 2 2 2
  spline S56 degree 2 poles (-13.6862, 3.3879) (-13.6036, 3.4657) (-13.3362, 3.5508) (-13.1307, 3.5508) knots 0 0 0 1 2 2 2
  spline S57 degree 2 poles (-13.1307, 3.5508) (-12.9448, 3.5508) (-12.6117, 3.467) (-12.5011, 3.3855) knots 0 0 0 1 2 2 2
  spline S58 degree 2 poles (-12.5011, 3.3855) (-12.3844, 3.2992) (-12.2616, 3.0561) (-12.2616, 2.8786) knots 0 0 0 1 2 2 2
  spline S59 degree 2 poles (-12.2616, 2.8786) (-12.2616, 2.8385) (-12.2701, 2.7473) (-12.2823, 2.7084) knots 0 0 0 1 2 2 2
  line L50 (-12.2823, 2.7084) -> (-12.4755, 2.7084)
  line L51 (-12.4755, 2.7084) -> (-12.4755, 2.7182)
  spline S60 degree 2 poles (-12.4755, 2.7182) (-12.461, 2.7437) (-12.4354, 2.8507) (-12.4354, 2.9054) knots 0 0 0 1 2 2 2
  spline S61 degree 2 poles (-12.4354, 2.9054) (-12.4354, 3.1023) (-12.6956, 3.3272) (-12.9362, 3.343) knots 0 0 0 1 2 2 2
  spline S62 degree 2 poles (-12.9362, 3.343) (-12.8815, 3.2627) (-12.8317, 3.1169) (-12.8317, 3.0306) knots 0 0 0 1 2 2 2
  spline S63 degree 2 poles (-12.8317, 3.0306) (-12.8317, 2.9479) (-12.8682, 2.8106) (-12.9204, 2.7413) knots 0 0 0 1 2 2 2
  spline S64 degree 2 poles (-12.9204, 2.7413) (-12.9824, 2.661) (-13.1708, 2.5784) (-13.3033, 2.5784) knots 0 0 0 1 2 2 2
  spline S65 degree 2 poles (-13.1757, 3.3478) (-13.3277, 3.3478) (-13.5197, 3.2919) (-13.572, 3.2421) knots 0 0 0 1 2 2 2
  spline S66 degree 2 poles (-13.572, 3.2421) (-13.6206, 3.1983) (-13.6571, 3.1072) (-13.6571, 3.0537) knots 0 0 0 1 2 2 2
  spline S67 degree 2 poles (-13.6571, 3.0537) (-13.6571, 2.9297) (-13.4796, 2.7826) (-13.3119, 2.7826) knots 0 0 0 1 2 2 2
  spline S68 degree 2 poles (-13.3119, 2.7826) (-13.217, 2.7826) (-13.0943, 2.8312) (-13.0505, 2.8847) knots 0 0 0 1 2 2 2
  spline S69 degree 2 poles (-13.0505, 2.8847) (-13.0189, 2.9236) (-12.9982, 3.0196) (-12.9982, 3.0755) knots 0 0 0 1 2 2 2
  spline S70 degree 2 poles (-12.9982, 3.0755) (-12.9982, 3.14) (-13.0432, 3.2883) (-13.0809, 3.3442) knots 0 0 0 1 2 2 2
  spline S71 degree 2 poles (-13.0809, 3.3442) (-13.0955, 3.3454) (-13.1453, 3.3478) (-13.1757, 3.3478) knots 0 0 0 1 2 2 2
  line L52 (-12.8062, 4.7105) -> (-12.8062, 4.5318)
  line L53 (-12.8062, 4.5318) -> (-12.2908, 4.5318)
  line L54 (-12.2908, 4.5318) -> (-12.2908, 4.3385)
  line L55 (-12.2908, 4.3385) -> (-12.8062, 4.3385)
  line L56 (-12.8062, 4.3385) -> (-12.8062, 3.676)
  line L57 (-12.8062, 3.676) -> (-13.0177, 3.676)
  line L58 (-13.0177, 3.676) -> (-13.7908, 4.347)
  line L59 (-13.7908, 4.347) -> (-13.7908, 4.5318)
  line L60 (-13.7908, 4.5318) -> (-12.9679, 4.5318)
  line L61 (-12.9679, 4.5318) -> (-12.9679, 4.7105)
  line L62 (-12.9679, 4.7105) -> (-12.8062, 4.7105)
  line L63 (-12.9679, 4.3385) -> (-13.5538, 4.3385)
  line L64 (-13.5538, 4.3385) -> (-12.9679, 3.8341)
  line L65 (-12.9679, 3.8341) -> (-12.9679, 4.3385)
  spline S72 degree 2 poles (-12.7673, 5.7802) (-12.6591, 5.7802) (-12.4743, 5.7109) (-12.4063, 5.6477) knots 0 0 0 1 2 2 2
  spline S73 degree 2 poles (-12.4063, 5.6477) (-12.3382, 5.5845) (-12.2592, 5.396) (-12.2592, 5.2794) knots 0 0 0 1 2 2 2
  spline S74 degree 2 poles (-12.2592, 5.2794) (-12.2592, 5.1724) (-12.3066, 4.9633) (-12.3443, 4.8867) knots 0 0 0 1 2 2 2
  line L66 (-12.3443, 4.8867) -> (-12.557, 4.8867)
  line L67 (-12.557, 4.8867) -> (-12.557, 4.9013)
  spline S75 degree 2 poles (-12.557, 4.9013) (-12.54, 4.9244) (-12.4962, 5.0107) (-12.4768, 5.063) knots 0 0 0 1 2 2 2
  spline S76 degree 2 poles (-12.4768, 5.063) (-12.4561, 5.1225) (-12.433, 5.221) (-12.433, 5.283) knots 0 0 0 1 2 2 2
  spline S77 degree 2 poles (-12.433, 5.283) (-12.433, 5.3438) (-12.4768, 5.458) (-12.5242, 5.4994) knots 0 0 0 1 2 2 2
  spline S78 degree 2 poles (-12.5242, 5.4994) (-12.5691, 5.5371) (-12.6883, 5.576) (-12.7685, 5.576) knots 0 0 0 1 2 2 2
  spline S79 degree 2 poles (-12.7685, 5.576) (-12.8487, 5.576) (-12.9508, 5.5322) (-12.9849, 5.4909) knots 0 0 0 1 2 2 2
  spline S80 degree 2 poles (-12.9849, 5.4909) (-13.0226, 5.4483) (-13.0542, 5.3219) (-13.0542, 5.2453) knots 0 0 0 1 2 2 2
  spline S81 degree 2 poles (-13.0542, 5.2453) (-13.0542, 5.1627) (-13.0286, 4.9986) (-13.0177, 4.9487) knots 0 0 0 1 2 2 2
  line L68 (-13.0177, 4.9487) -> (-13.7908, 4.9487)
  line L69 (-13.7908, 4.9487) -> (-13.7908, 5.7717)
  line L70 (-13.7908, 5.7717) -> (-13.6145, 5.7717)
  line L71 (-13.6145, 5.7717) -> (-13.6145, 5.142)
  line L72 (-13.6145, 5.142) -> (-13.2146, 5.142)
  spline S82 degree 2 poles (-13.2146, 5.142) (-13.2195, 5.1785) (-13.2231, 5.249) (-13.2231, 5.2781) knots 0 0 0 1 2 2 2
  spline S83 degree 2 poles (-13.2231, 5.2781) (-13.2231, 5.3936) (-13.1854, 5.5529) (-13.1295, 5.6258) knots 0 0 0 1 2 2 2
  spline S84 degree 2 poles (-13.1295, 5.6258) (-13.0736, 5.6999) (-12.9034, 5.7802) (-12.7673, 5.7802) knots 0 0 0 1 2 2 2
  point P0 (0, 0)
  constraints: 2 other
extrude "Extrusion7" add sketch "Sketch7" along normal blind 0.1 bodies 5
sketch "Sketch8" plane through (-14.5, 6.05, 1.1) normal (0, 1, 0) x (1, 0, 0)
  line L0 (0, 0) -> (-4.5, 0)
  line L1 (0, -1.5) -> (-4.5, -1.5)
  arc A0 (-4.5, 0) -> (-4.5, -1.5) centre (-4.5, -0.75) ccw
  line L2 (0, -1.1979) -> (-4.5, -1.1979)
  arc A1 (-4.5, -0.3021) -> (-4.5, -1.1979) centre (-4.5, -0.75) ccw
  line L3 (-4.5, -0.3021) -> (0, -0.3021)
  line L4 (0, -1.5) -> (0, -1.1979)
  line L5 (0, -0.3021) -> (0, 0)
  line L6 (33.3, 0) -> (-4.3, 0)
  point P0 (14.5, 1.1)
  constraints: 12 end point, 4 point on circle, 2 centre point, 1 horizontal, 1 perpendicular, 2 other
extrude "Extrusion8" add sketch "Sketch8" against normal blind 7.6 separate body
sketch "Sketch9" plane through (-14.5, 6.05, 1.1) normal (0, 1, 0) x (1, 0, 0)
  line L0 (0, 0) -> (-4.5, 0)
  arc A0 (-4.5, 0) -> (-4.5, -1.5) centre (-4.5, -0.75) ccw
  line L1 (-4.5, -1.5) -> (0, -1.5)
  line L2 (0, -1.5) -> (0, -1.1979)
  line L3 (0, -1.1979) -> (-4.5, -1.1979)
  arc A1 (-4.5, -0.3021) -> (-4.5, -1.1979) centre (-4.5, -0.75) ccw
  line L4 (-4.5, -0.3021) -> (0, -0.3021)
  line L5 (0, -0.3021) -> (0, 0)
  point P0 (14.5, 1.1)
extrude "Extrusion9" cut sketch "Sketch9" against normal blind 0.2 bodies 7
sketch "Sketch10" plane through (0, 0, 0) normal (0, 0, -1) x (-1, 0, 0)
  line L0 (18.8, 6.05) -> (18.8, -6.05)
  line L1 (5.6, -4.98) -> (3.7, -4.98)
  line L2 (3.7, -4.98) -> (3.7, -5.78)
  line L3 (3.7, -5.78) -> (5.6, -5.78)
  line L4 (5.6, -5.78) -> (5.6, -4.98)
  line L5 (5.6, -3.64) -> (3.7, -3.64)
  line L6 (3.7, -3.64) -> (3.7, -4.44)
  line L7 (3.7, -4.44) -> (5.6, -4.44)
  line L8 (5.6, -4.44) -> (5.6, -3.64)
  line L9 (5.6, -2.3) -> (3.7, -2.3)
  line L10 (3.7, -2.3) -> (3.7, -3.1)
  line L11 (3.7, -3.1) -> (5.6, -3.1)
  line L12 (5.6, -3.1) -> (5.6, -2.3)
  line L13 (5.6, -0.96) -> (3.7, -0.96)
  line L14 (3.7, -0.96) -> (3.7, -1.76)
  line L15 (3.7, -1.76) -> (5.6, -1.76)
  line L16 (5.6, -1.76) -> (5.6, -0.96)
  line L17 (5.6, 0.38) -> (3.7, 0.38)
  line L18 (3.7, 0.38) -> (3.7, -0.42)
  line L19 (3.7, -0.42) -> (5.6, -0.42)
  line L20 (5.6, -0.42) -> (5.6, 0.38)
  line L21 (5.6, 1.72) -> (3.7, 1.72)
  line L22 (3.7, 1.72) -> (3.7, 0.92)
  line L23 (3.7, 0.92) -> (5.6, 0.92)
  line L24 (5.6, 0.92) -> (5.6, 1.72)
  line L25 (5.6, 3.06) -> (3.7, 3.06)
  line L26 (3.7, 3.06) -> (3.7, 2.26)
  line L27 (3.7, 2.26) -> (5.6, 2.26)
  line L28 (5.6, 2.26) -> (5.6, 3.06)
  line L29 (5.6, 4.4) -> (3.7, 4.4)
  line L30 (3.7, 4.4) -> (3.7, 3.6)
  line L31 (3.7, 3.6) -> (5.6, 3.6)
  line L32 (5.6, 3.6) -> (5.6, 4.4)
  line L33 (5.6, 5.76) -> (3.7, 5.76)
  line L34 (3.7, 5.76) -> (3.7, 4.96)
  line L35 (3.7, 4.96) -> (5.6, 4.96)
  line L36 (5.6, 4.96) -> (5.6, 5.76)
  point P0 (0, 0)
  dimension "d82" = 0.8
  dimension "d83" = 0.8
  dimension "d84" = 0.8
  dimension "d85" = 0.8
  dimension "d86" = 0.8
  dimension "d87" = 0.8
  dimension "d88" = 0.8
  dimension "d89" = 0.8
  dimension "d90" = 0.8
  constraints: 72 end point, 18 parallel, 9 perpendicular
  measures "d82" distance of L2.end L1.end
  measures "d83" distance of L7.start L5.end
  measures "d84" distance of L11.start L9.end
  measures "d85" distance of L15.start L13.end
  measures "d86" distance of L19.start L17.end
  measures "d87" distance of L23.start L21.end
  measures "d88" distance of L27.start L25.end
  measures "d89" distance of L31.start L29.end
  measures "d90" distance of L35.start L33.end
extrude "Extrusion10" add sketch "Sketch10" along normal blind 1 separate body
chamfer "Chamfer3" distance 0.09 angle 45 36 edges at (-4.65, 5.76, -1) (-4.65, 4.96, -1) (-5.6, 5.36, -1) (-3.7, 5.36, -1) (-4.65, 4.4, -1) (-4.65, 3.6, -1) (-5.6, 4, -1) (-3.7, 4, -1) (-5.6, 2.66, -1) (-4.65, 3.06, -1) (-3.7, 2.66, -1) (-4.65, 2.26, -1) (-4.65, 1.72, -1) (-5.6, 1.32, -1) (-4.65, 0.92, -1) (-3.7, 1.32, -1) (-4.65, 0.38, -1) (-3.7, -0.02, -1) (-5.6, -0.02, -1) (-4.65, -0.42, -1) (-4.65, -0.96, -1) (-5.6, -1.36, -1) (-4.65, -1.76, -1) (-3.7, -1.36, -1) (-4.65, -2.3, -1) (-3.7, -2.7, -1) (-4.65, -3.1, -1) (-5.6, -2.7, -1) (-4.65, -3.64, -1) (-3.7, -4.04, -1) (-4.65, -4.44, -1) (-5.6, -4.04, -1) (-4.65, -4.98, -1) (-3.7, -5.38, -1) (-4.65, -5.78, -1) (-5.6, -5.38, -1)